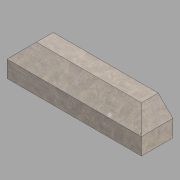
# Autodesk Inventor part: Return_L
Saved by Autodesk Inventor 2022.2 (Build 262287000, 287)
## iProperties
Created: 2021-12-31
Part Number: Return_L
Material: Limestone
Document SubType Name: Modeling
Designer: awelt
Density: 2.6 g/cm^3
Appearance: Kasota Gray
Mass: 41364.6 g
Surface Area: 4121.24 cm^2
Volume: 15909.4 cm^3
Author: awelt
Autodesk Inventor part; units mm, degrees
ref_plane "YZ Plane" through (0, 0, 0) normal (1, 0, 0) x (0, 1, 0)
ref_plane "XZ Plane" through (0, 0, 0) normal (0, 1, 0) x (-1, 0, 0)
ref_plane "XY Plane" through (0, 0, 0) normal (0, 0, 1) x (1, 0, 0)
sketch "Sketch1" plane through (0, 0, 0) normal (1, 0, 0) x (0, 1, 0)
  line L0 (0, 0) -> (190.5, 0)
  line L1 (0, 0) -> (0, 190.5)
  line L2 (0, 190.5) -> (101.6, 190.5)
  line L3 (190.5, 0) -> (190.5, 101.6)
  line L4 (190.5, 101.6) -> (101.6, 190.5)
  dimension "d0" = 190.5
  dimension "d1" = 190.5
  dimension "d2" = 101.6
  dimension "d3" = 101.6
  dimension "d4" = 88.9
  dimension "d5" = 88.9
  constraints: 10 end point, 2 vertical, 1 horizontal, 1 perpendicular
  measures "d0" distance of L0.start L0.end
  measures "d1" distance of L0.start L1.end
  measures "d2" distance of L1.end L2.end
  measures "d3" distance of L0.end L3.end
  measures "d4" horizontal distance of L2.end L3.end
  measures "d5" horizontal distance of L2.end L3.end
extrude "Extrusion1" add sketch "Sketch1" along normal blind 406.4
sketch "Sketch2" plane through (0, 0, 190.5) normal (0, 0, 1) x (1, 0, 0)
  line L0 (0, 0) -> (0, 190.5) projected
  line L1 (0, 190.5) -> (88.9, 190.5)
  line L2 (0, 190.5) -> (406.4, 190.5) projected
  line L3 (0, 190.5) -> (0, 101.6)
  line L4 (0, 101.6) -> (88.9, 190.5)
  dimension "d8" = 88.9
  dimension "d9" = 88.9
  constraints: 6 end point, 2 point on line
  measures "d8" distance of L0.end L1.end
  measures "d9" distance of L0.end L3.end
extrude "Extrusion2" cut sketch "Sketch2" against normal up to surface (190.5 mm away)
mirror "Mirror1" about plane through (406.4, 95.25, 95.25) normal (1, 0, 0) of "Extrusion1", "Extrusion2"
body "Solid1"
